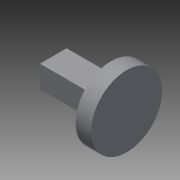
# Autodesk Inventor part: Motor
Saved by Autodesk Inventor 2015 (Build 190159000, 159)
## iProperties
Created: 2015-04-05
Part Number: Motor
Material: Generic
Document SubType Name: Modeling
Designer: Jesse
Density: 1 g/cm^3
Appearance: Default
Author: Jesse
Autodesk Inventor part; units mm, degrees
ref_plane "YZ Plane" through (0, 0, 0) normal (1, 0, 0) x (0, 1, 0)
ref_plane "XZ Plane" through (0, 0, 0) normal (0, 1, 0) x (-1, 0, 0)
ref_plane "XY Plane" through (0, 0, 0) normal (0, 0, 1) x (1, 0, 0)
sketch "Sketch1" plane through (0, 0, 0) normal (0, 1, 0) x (-1, 0, 0)
  line L0 (13, 6) -> (-13, 6)
  line L1 (-13, 6) -> (-13, -6)
  line L2 (-13, -6) -> (13, -6)
  line L3 (13, -6) -> (13, 6)
  point P0 (0, 0)
  dimension "d0" = 6
  dimension "d1" = 6
  dimension "d2" = 26
  dimension "d3" = 13
  constraints: 8 end point, 2 parallel, 1 horizontal, 1 perpendicular
  measures "d0" distance from line of L2 point (0, 0)
  measures "d1" distance from line of point (0, 0) L0
  measures "d2" distance between parallel lines of L3 L1
  measures "d3" distance from line of L1 point (0, 0)
extrude "Extrusion1" add sketch "Sketch1" along normal blind 10
sketch "Sketch2" plane through (13, 0, 6) normal (1, 0, 0) x (0, 0, -1)
  line L0 (0, 10) -> (0, 0)
  circle A0 centre (6, 5) radius 16
  point P0 (6, 0)
  dimension "d6" = 32
  constraints: 2 end point, 1 centre point, 1 vertical
  measures "d6" diameter of A0
extrude "Extrusion2" add sketch "Sketch2" along normal blind 7
body "Solid1"
